Autodesk Inventor part; units mm, degrees
(part 2 of 2)
  spline S285 degree 2 poles (-38.0768, -6.3531) (-38.0768, -6.7545) (-38.1262, -7.2917) (-38.2065, -7.5016) knots 0 0 0 1 2 2 2
  spline S286 degree 2 poles (-38.2065, -7.5016) (-38.2806, -7.6992) (-38.5554, -7.9123) (-38.7777, -7.9123) knots 0 0 0 1 2 2 2
  spline S287 degree 2 poles (-38.7777, -7.9123) (-38.9877, -7.9123) (-39.2625, -7.7116) (-39.3396, -7.5109) knots 0 0 0 1 2 2 2
  spline S288 degree 2 poles (-41.5102, -4.8062) (-41.3712, -4.8062) (-41.0964, -4.8742) (-40.9637, -4.9267) knots 0 0 0 1 2 2 2
  spline S289 degree 2 poles (-40.9637, -4.9267) (-40.8402, -4.9791) (-40.658, -5.0903) (-40.587, -5.1397) knots 0 0 0 1 2 2 2
  line L229 (-40.587, -5.1397) -> (-40.5561, -5.1397)
  line L230 (-40.5561, -5.1397) -> (-40.5561, -4.5994)
  spline S290 degree 2 poles (-40.5561, -4.5994) (-40.7228, -4.5098) (-41.294, -4.3647) (-41.5503, -4.3647) knots 0 0 0 1 2 2 2
  spline S291 degree 2 poles (-41.5503, -4.3647) (-41.8097, -4.3647) (-42.1956, -4.4697) (-42.3531, -4.5809) knots 0 0 0 1 2 2 2
  spline S292 degree 2 poles (-42.3531, -4.5809) (-42.5198, -4.7013) (-42.6927, -5.0502) (-42.6927, -5.2848) knots 0 0 0 1 2 2 2
  spline S293 degree 2 poles (-42.6927, -5.2848) (-42.6927, -5.5997) (-42.279, -6.0752) (-41.9887, -6.137) knots 0 0 0 1 2 2 2
  line L231 (-41.9887, -6.137) -> (-41.9887, -6.174)
  spline S294 degree 2 poles (-41.9887, -6.174) (-42.1091, -6.1987) (-42.3839, -6.3099) (-42.5013, -6.421) knots 0 0 0 1 2 2 2
  spline S295 degree 2 poles (-42.5013, -6.421) (-42.6186, -6.5291) (-42.7668, -6.8749) (-42.7668, -7.125) knots 0 0 0 1 2 2 2
  spline S296 degree 2 poles (-42.7668, -7.125) (-42.7668, -7.3812) (-42.5908, -7.8166) (-42.4302, -7.9833) knots 0 0 0 1 2 2 2
  spline S297 degree 2 poles (-42.4302, -7.9833) (-42.2635, -8.1562) (-41.7911, -8.3353) (-41.4916, -8.3353) knots 0 0 0 1 2 2 2
  spline S298 degree 2 poles (-41.4916, -8.3353) (-41.2045, -8.3353) (-40.6426, -8.1963) (-40.4511, -8.1006) knots 0 0 0 1 2 2 2
  line L232 (-40.4511, -8.1006) -> (-40.4511, -7.5603)
  line L233 (-40.4511, -7.5603) -> (-40.4882, -7.5603)
  spline S299 degree 2 poles (-40.4882, -7.5603) (-40.6487, -7.6776) (-41.1922, -7.8938) (-41.4608, -7.8938) knots 0 0 0 1 2 2 2
  spline S300 degree 2 poles (-41.4608, -7.8938) (-41.6182, -7.8938) (-41.9332, -7.795) (-42.0381, -7.6807) knots 0 0 0 1 2 2 2
  spline S301 degree 2 poles (-42.0381, -7.6807) (-42.14, -7.5665) (-42.2481, -7.2948) (-42.2481, -7.0879) knots 0 0 0 1 2 2 2
  spline S302 degree 2 poles (-42.2481, -7.0879) (-42.2481, -6.8811) (-42.1277, -6.6124) (-42.0196, -6.5353) knots 0 0 0 1 2 2 2
  spline S303 degree 2 poles (-42.0196, -6.5353) (-41.9115, -6.4581) (-41.6182, -6.3994) (-41.4453, -6.3994) knots 0 0 0 1 2 2 2
  line L234 (-41.4453, -6.3994) -> (-41.2292, -6.3994)
  line L235 (-41.2292, -6.3994) -> (-41.2292, -5.9764)
  line L236 (-41.2292, -5.9764) -> (-41.399, -5.9764)
  spline S304 degree 2 poles (-41.399, -5.9764) (-41.7417, -5.9764) (-42.174, -5.6491) (-42.174, -5.3373) knots 0 0 0 1 2 2 2
  spline S305 degree 2 poles (-42.174, -5.3373) (-42.174, -5.1922) (-42.0628, -4.9853) (-41.9733, -4.9236) knots 0 0 0 1 2 2 2
  spline S306 degree 2 poles (-41.9733, -4.9236) (-41.8776, -4.8587) (-41.6429, -4.8062) (-41.5102, -4.8062) knots 0 0 0 1 2 2 2
  spline S307 degree 2 poles (-47.4938, -5.5936) (-47.4938, -5.8406) (-47.3178, -6.2852) (-47.1603, -6.4395) knots 0 0 0 1 2 2 2
  spline S308 degree 2 poles (-47.1603, -6.4395) (-46.9627, -6.6341) (-46.4286, -6.8347) (-46.021, -6.8347) knots 0 0 0 1 2 2 2
  line L237 (-46.021, -6.8347) -> (-45.5919, -6.8347)
  line L238 (-45.5919, -6.8347) -> (-45.5919, -8.255)
  line L239 (-45.5919, -8.255) -> (-45.0855, -8.255)
  line L240 (-45.0855, -8.255) -> (-45.0855, -4.445)
  line L241 (-45.0855, -4.445) -> (-46.0426, -4.445)
  spline S309 degree 2 poles (-46.0426, -4.445) (-46.3823, -4.445) (-46.8578, -4.5562) (-47.0399, -4.6827) knots 0 0 0 1 2 2 2
  spline S310 degree 2 poles (-47.0399, -4.6827) (-47.253, -4.8279) (-47.4938, -5.2755) (-47.4938, -5.5936) knots 0 0 0 1 2 2 2
  spline S311 degree 2 poles (-46.9658, -5.609) (-46.9658, -5.4114) (-46.83, -5.1212) (-46.691, -5.0285) knots 0 0 0 1 2 2 2
  spline S312 degree 2 poles (-46.691, -5.0285) (-46.5706, -4.9483) (-46.2495, -4.8834) (-46.0118, -4.8834) knots 0 0 0 1 2 2 2
  line L242 (-46.0118, -4.8834) -> (-45.5919, -4.8834)
  line L243 (-45.5919, -4.8834) -> (-45.5919, -6.4025)
  line L244 (-45.5919, -6.4025) -> (-45.9377, -6.4025)
  spline S313 degree 2 poles (-45.9377, -6.4025) (-46.2464, -6.4025) (-46.6262, -6.3037) (-46.7497, -6.174) knots 0 0 0 1 2 2 2
  spline S314 degree 2 poles (-46.7497, -6.174) (-46.8639, -6.0598) (-46.9658, -5.7912) (-46.9658, -5.609) knots 0 0 0 1 2 2 2
  line L245 (-50.7388, -4.445) -> (-49.4266, -8.255)
  line L246 (-49.4266, -8.255) -> (-48.8801, -8.255)
  line L247 (-48.8801, -8.255) -> (-47.5679, -4.445)
  line L248 (-47.5679, -4.445) -> (-48.1113, -4.445)
  line L249 (-48.1113, -4.445) -> (-49.1672, -7.6097)
  line L250 (-49.1672, -7.6097) -> (-50.2231, -4.445)
  line L251 (-50.2231, -4.445) -> (-50.7388, -4.445)
  spline S315 degree 2 poles (-53.4095, -6.35) (-53.4095, -7.3751) (-52.8136, -8.3353) (-52.193, -8.3353) knots 0 0 0 1 2 2 2
  spline S316 degree 2 poles (-52.193, -8.3353) (-51.5631, -8.3353) (-50.9734, -7.3565) (-50.9734, -6.3531) knots 0 0 0 1 2 2 2
  spline S317 degree 2 poles (-50.9734, -6.3531) (-50.9734, -5.3219) (-51.5693, -4.3678) (-52.193, -4.3678) knots 0 0 0 1 2 2 2
  spline S318 degree 2 poles (-52.193, -4.3678) (-52.8198, -4.3678) (-53.4095, -5.3558) (-53.4095, -6.35) knots 0 0 0 1 2 2 2
  spline S319 degree 2 poles (-52.7549, -7.5109) (-52.829, -7.3226) (-52.8908, -6.7421) (-52.8908, -6.35) knots 0 0 0 1 2 2 2
  spline S320 degree 2 poles (-52.8908, -6.35) (-52.8908, -5.9579) (-52.829, -5.3805) (-52.7518, -5.186) knots 0 0 0 1 2 2 2
  spline S321 degree 2 poles (-52.7518, -5.186) (-52.6746, -4.9915) (-52.406, -4.7908) (-52.193, -4.7908) knots 0 0 0 1 2 2 2
  spline S322 degree 2 poles (-52.193, -4.7908) (-51.9799, -4.7908) (-51.7052, -4.9915) (-51.6249, -5.1922) knots 0 0 0 1 2 2 2
  spline S323 degree 2 poles (-51.6249, -5.1922) (-51.5477, -5.3867) (-51.4921, -5.9795) (-51.4921, -6.3531) knots 0 0 0 1 2 2 2
  spline S324 degree 2 poles (-51.4921, -6.3531) (-51.4921, -6.7545) (-51.5415, -7.2917) (-51.6218, -7.5016) knots 0 0 0 1 2 2 2
  spline S325 degree 2 poles (-51.6218, -7.5016) (-51.6959, -7.6992) (-51.9707, -7.9123) (-52.193, -7.9123) knots 0 0 0 1 2 2 2
  spline S326 degree 2 poles (-52.193, -7.9123) (-52.4029, -7.9123) (-52.6777, -7.7116) (-52.7549, -7.5109) knots 0 0 0 1 2 2 2
  line L252 (-56.0555, -8.255) -> (-54.1968, -8.255)
  line L253 (-54.1968, -8.255) -> (-54.1968, -7.866)
  line L254 (-54.1968, -7.866) -> (-54.8884, -7.866)
  line L255 (-54.8884, -7.866) -> (-54.8884, -5.3126)
  line L256 (-54.8884, -5.3126) -> (-54.1968, -5.3126)
  line L257 (-54.1968, -5.3126) -> (-54.1968, -4.9637)
  spline S327 degree 2 poles (-54.1968, -4.9637) (-54.5889, -4.9637) (-54.9594, -4.7414) (-54.9841, -4.4326) knots 0 0 0 1 2 2 2
  line L258 (-54.9841, -4.4326) -> (-55.3793, -4.4326)
  line L259 (-55.3793, -4.4326) -> (-55.3793, -7.866)
  line L260 (-55.3793, -7.866) -> (-56.0555, -7.866)
  line L261 (-56.0555, -7.866) -> (-56.0555, -8.255)
  point P0 (0, 31.75)
  constraints: 2 end point, 2 midpoint, 1 horizontal
emboss "Emboss2" sketch "Sketch8" operation cut depth 2.54 direction (0, -1, 0) wrap yes faces at (-22.0263, -1.7782, -40.2167)
sketch "Sketch9" plane through (0, 0, -12.7) normal (0, 0, 1) x (1, 0, 0)
  line L0 (3.6662, 6.35) -> (7.3323, 0)
  line L1 (7.3323, 0) -> (3.6662, -6.35)
  line L2 (3.6662, -6.35) -> (-3.6662, -6.35)
  line L3 (-3.6662, -6.35) -> (-7.3323, 0)
  line L4 (-7.3323, 0) -> (-3.6662, 6.35)
  line L5 (-3.6662, 6.35) -> (3.6662, 6.35)
  line L6 (3.6662, 6.35) -> (-3.6662, 6.35) projected
  point P0 (0, 0)
  point P1 (0, 0)
  constraints: 12 end point, 1 coincident, 1 collinear, 13 other
extrude "Extrusion4" cut sketch "Sketch9" along normal blind 25.4
sketch "Sketch10" plane through (0, 0, -44.45) normal (0, 0, -1) x (-1, 0, 0)
  line L0 (3.7395, 6.477) -> (7.479, 0)
  line L1 (7.479, 0) -> (3.7395, -6.477)
  line L2 (3.7395, -6.477) -> (-3.7395, -6.477)
  line L3 (-3.7395, -6.477) -> (-7.479, 0)
  line L4 (-7.479, 0) -> (-3.7395, 6.477)
  line L5 (-3.7395, 6.477) -> (3.7395, 6.477)
  point P0 (0, 0)
  point P1 (0, 0)
  dimension "d32" = 12.954
  constraints: 12 end point, 1 coincident, 1 horizontal, 13 other
  measures "d32" distance between parallel lines of L2 L5
extrude "Extrusion5" cut sketch "Sketch10" against normal through all
sketch "Sketch11" plane through (0, 0, -12.7) normal (0, 0, 1) x (1, 0, 0)
  line L0 (7.479, 0) -> (3.7395, 6.477) projected
  line L1 (7.479, 0) -> (3.7395, -6.477)
  line L2 (3.7395, -6.477) -> (-3.7395, -6.477)
  line L3 (-3.7395, -6.477) -> (-7.479, 0)
  line L4 (-7.479, 0) -> (-3.7395, 6.477)
  line L5 (-3.7395, 6.477) -> (3.7395, 6.477)
  line L6 (3.7395, 6.477) -> (7.479, 0)
  circle A0 centre (0, 0) radius 15.748
  constraints: 12 end point, 2 coincident, 1 centre point, 13 other
extrude "Extrusion6" add sketch "Sketch11" along normal blind 19.05
equation "\"d0\" = printedHexSize"
equation "\"d1\" = lengthOfHexExtrusion"
equation "\"hexSize\" = 12.7"
equation "\"slipFitOffset\" = 0"
equation "\"printedHexSize\" = hexSize - slipFitOffset"
equation "\"lengthOfHexExtrusion\" = 25.4"
equation "\"bushingSlipOffset\" = 0.381"
body "Solid1"
